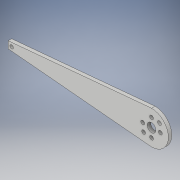
# Autodesk Inventor part: ClawLinkage
Saved by Autodesk Inventor 2017 (Build 210142000, 142)
## iProperties
Created: 2017-09-29
Part Number: ClawLinkage
Material: Generic
Document SubType Name: Modeling
Designer: User
Density: 1 g/cm^3
Appearance: Default
Author: User
Autodesk Inventor part; units mm, degrees
ref_plane "YZ Plane" through (0, 0, 0) normal (1, 0, 0) x (0, 1, 0)
ref_plane "XZ Plane" through (0, 0, 0) normal (0, 1, 0) x (-1, 0, 0)
ref_plane "XY Plane" through (0, 0, 0) normal (0, 0, 1) x (1, 0, 0)
sketch "Sketch1" plane through (0, 0, 0) normal (0, 0, 1) x (1, 0, 0)
  circle A0 centre (0, 0) radius 15.24
  line L0 (0, 0) -> (-8.001, 0)
  line L1 (0, 0) -> (8.001, 0)
  line L2 (0, 0) -> (0, 8.001)
  line L3 (0, 0) -> (0, -8.001)
  circle A1 centre (8.001, 0) radius 1.7526
  circle A2 centre (0, 8.001) radius 1.7526
  circle A3 centre (-8.001, 0) radius 1.7526
  circle A4 centre (0, -8.001) radius 1.7526
  dimension "d0" = 30.48
  dimension "d11" = 8.001
  dimension "d12" = 8.001
  dimension "d13" = 8.001
  dimension "d14" = 8.001
  dimension "d15" = 3.5052
  dimension "d16" = 3.5052
  dimension "d17" = 3.5052
  dimension "d18" = 3.5052
  constraints: 8 end point, 5 centre point, 5 coincident, 2 horizontal, 2 vertical
  measures "d0" diameter of A0
  measures "d11" distance of L0.start L0.end
  measures "d12" distance of L0.start L1.end
  measures "d13" distance of L0.start L2.end
  measures "d14" distance of L0.start L3.end
  measures "d15" diameter of A1
  measures "d16" diameter of A2
  measures "d17" diameter of A3
  measures "d18" diameter of A4
extrude "Extrusion1" add sketch "Sketch1" along normal blind 3.175 contours A0 | A1 | A2 | A3 | A4
sketch "Sketch2" plane through (0, 0, 3.175) normal (0, 0, 1) x (1, 0, 0)
  circle A0 centre (0, 0) radius 15.24 projected
  line L0 (-15.24, 0) -> (-15.24, 3.175)
  line L1 (-15.24, 0) -> (-15.24, -3.175)
  dimension "d3" = 3.175
  dimension "d4" = 3.175
  constraints: 4 end point, 4 vertical, 1 horizontal alignment, 1 other
  measures "d3" distance of L0.start L0.end
  measures "d4" distance of L0.start L1.end
ref_plane "Work Plane1" through (-15.24, 0, 3.175) normal (1, 0, 0) x (0, 1, 0)
sketch "Sketch3" plane through (-15.24, 0, 3.175) normal (1, 0, 0) x (0, 1, 0)
  line L0 (15.24, 0) -> (-15.24, 0) projected
  line L1 (-15.24, -3.175) -> (15.24, -3.175) projected
  line L2 (0, -3.175) -> (3.175, -3.175)
  line L3 (3.175, -3.175) -> (3.175, 0)
  line L4 (3.175, 0) -> (-3.175, 0)
  line L5 (-3.175, 0) -> (-3.175, -3.175)
  line L6 (-3.175, -3.175) -> (3.175, -3.175)
  dimension "d6" = 6.35
  constraints: 10 end point, 3 perpendicular, 1 collinear, 1 point on line
  measures "d6" distance of L3.end L4.end
extrude "Extrusion2" add sketch "Sketch3" against normal blind 115.0493
sketch "Sketch4" plane through (-15.24, 0, 3.175) normal (1, 0, 0) x (0, 0, -1)
  line L0 (3.175, -3.175) -> (3.175, 0) projected
  line L1 (0, 3.175) -> (3.175, 3.175)
  line L2 (3.175, 3.175) -> (3.175, -3.175)
  line L3 (3.175, -3.175) -> (0, -3.175)
  line L4 (0, -3.175) -> (0, 3.175)
  constraints: 8 end point, 2 parallel, 1 horizontal, 1 perpendicular
extrude "Extrusion3" add sketch "Sketch4" along normal blind 12.7
extrude "Extrusion4" cut sketch "Sketch1" along normal blind 12.7 contours A1 | A2 | A3 | A4
sketch "Sketch5" plane through (0, 0, 0) normal (0, 0, -1) x (-1, 0, 0)
  circle A0 centre (0, 0) radius 3.9878
  dimension "d21" = 7.9756
  constraints: 1 centre point, 1 coincident
  measures "d21" diameter of A0
extrude "Extrusion5" cut sketch "Sketch5" against normal blind 12.7
sketch "Sketch7" plane through (0, 0, 3.175) normal (0, 0, 1) x (1, 0, 0)
  line L0 (-130.2893, -3.175) -> (-130.2893, 3.175) projected
  line L1 (-130.2893, 0) -> (-127.1143, 0)
  circle A0 centre (-127.1143, 0) radius 1.5875
  point P0 (0, 0)
  dimension "d26" = 3.175
  dimension "d27" = 3.175
  constraints: 2 end point, 1 centre point, 1 coincident, 1 horizontal, 1 midpoint
  measures "d26" distance of L1.start L1.end
  measures "d27" diameter of A0
extrude "Extrusion7" cut sketch "Sketch7" against normal blind 3.175
sketch "Sketch9" plane through (0, 0, 3.175) normal (0, 0, 1) x (1, 0, 0)
  line L0 (0, 0) -> (7.1842, 7.1842)
  line L1 (0, 0) -> (10.16, 0) construction
  line L2 (0, 0) -> (-7.1842, -7.1842)
  circle A0 centre (-7.1842, -7.1842) radius 1.7526
  circle A1 centre (7.1842, 7.1842) radius 1.7526
  dimension "d37" = 10.16
  dimension "d38" = 45
  dimension "d39" = 10.16
  dimension "d40" = 3.5052
  dimension "d41" = 3.5052
  constraints: 6 end point, 2 centre point, 2 coincident, 1 equal length, 1 horizontal
  measures "d37" distance of L0.start L0.end
  measures "d38" angle of L1 L0
  measures "d39" distance of L0.start L2.end
  measures "d40" diameter of A0
  measures "d41" diameter of A1
extrude "Extrusion9" cut sketch "Sketch9" against normal blind 25.4
sketch "Sketch11" plane through (0, 0, 3.175) normal (0, 0, 1) x (1, 0, 0)
  line L0 (-130.2893, 3.175) -> (0, 15.24)
  arc A0 (-14.9056, -3.175) -> (-14.9056, 3.175) centre (0, 0) ccw projected
  line L1 (0, -15.24) -> (-130.2893, -3.175)
  arc A1 (-14.9056, -3.175) -> (-14.9056, 3.175) centre (0, 0) ccw projected
  constraints: 4 end point, 2 point on circle
extrude "Extrusion11" cut sketch "Sketch11" against normal blind 25.4 fills toward (-65.1493, 9.2573) open curves L0
extrude "Extrusion12" cut sketch "Sketch11" against normal blind 25.4 fills toward (-65.1493, -9.2573) open curves L1
sketch "Sketch12" plane through (0, 0, 3.175) normal (0, 0, 1) x (1, 0, 0)
  line L0 (-14.9056, 3.175) -> (-130.2893, 3.175) projected
  arc A0 (-2.7985, 14.9809) -> (-14.9056, 3.175) centre (0, 0) ccw projected
  line L1 (-130.2893, 3.175) -> (-2.7985, 14.9809)
  line L2 (-2.7985, 14.9809) -> (0, 15.24) projected
  arc A1 (-2.7985, 14.9809) -> (-14.9056, 3.175) centre (0, 0) ccw
  arc A2 (-14.9056, -3.175) -> (-2.7985, -14.9809) centre (0, 0) ccw projected
  arc A3 (-2.7985, -14.9809) -> (-14.9056, -3.175) centre (0, 0) ccw
  line L3 (-130.2893, -3.175) -> (-14.9056, -3.175) projected
  line L4 (-130.2893, -3.175) -> (-14.9056, -3.175)
  line L5 (-14.9056, -3.175) -> (-14.9056, 3.175)
  line L6 (-130.2893, 3.175) -> (-14.9056, 3.175)
  arc A4 (0, -15.24) -> (0, 15.24) centre (0, 0) ccw projected
  line L7 (-130.2893, -3.175) -> (0, -15.24)
  arc A5 (-14.9056, -3.175) -> (-2.7985, -14.9809) centre (0, 0) ccw
  line L8 (-2.7985, -14.9809) -> (0, -15.24) projected
  arc A6 (-14.9056, -3.175) -> (-2.7985, -14.9809) centre (0, 0) ccw
  constraints: 10 end point, 9 point on circle, 4 centre point, 2 coincident, 2 perpendicular, 1 collinear, 1 concentric
extrude "Extrusion13" add sketch "Sketch12" against normal blind 3.175 contours A2 L7 L3
extrude "Extrusion14" add sketch "Sketch12" against normal blind 3.175 contours L0 L1 A0
body "Solid1"
